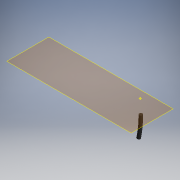
# Autodesk Inventor part: wire
Saved by Autodesk Inventor 2018 (Build 220112000, 112)
## iProperties
Created: 2018-02-17
Part Number: wire
Material: Generic
Document SubType Name: Modeling
Designer: artur
Density: 1 g/cm^3
Appearance: Default
Author: artur
Autodesk Inventor part; units mm, degrees
ref_plane "YZ Plane" through (0, 0, 0) normal (1, 0, 0) x (0, 1, 0)
ref_plane "XY Plane" through (0, 0, 0) normal (0, 0, 1) x (1, 0, 0)
sketch "Sketch1" plane through (0, 0, 0) normal (0, 0, 1) x (1, 0, 0)
  arc A0 (-4.243, -68.3065) -> (0, -26.034) centre (-201.1874, -27.1897) ccw
  point P0 (0, 0)
  constraints: 2 point on circle, 1 centre point
ref_plane "Work Plane1" through (0, -26.034, 0) normal (0, 1, 0) x (-1, 0, 0)
sketch "Sketch2" plane through (0, -26.034, 0) normal (0, 1, 0) x (-1, 0, 0)
  circle A0 centre (0, 0) radius 3.175
  dimension "d0" = 6.35
  constraints: 1 centre point, 1 coincident
  measures "d0" diameter of A0
sweep "Sweep1" add profiles "Sketch2" path "Sketch1"
body "Solid1"
